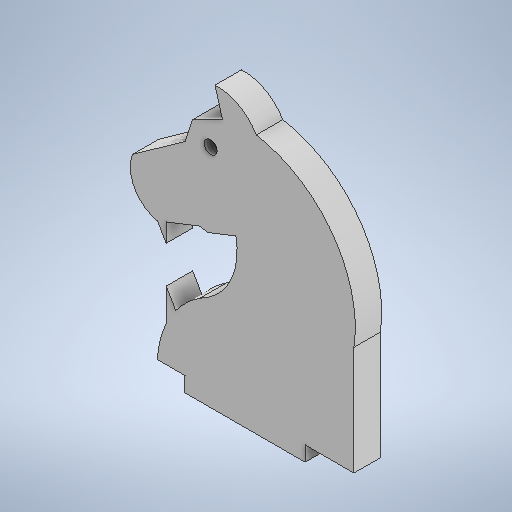
# Autodesk Inventor part: KIGTH TOP ABREBOTELLA 1.2
Saved by Autodesk Inventor 2025.1 (Build 291241000, 241)
## iProperties
Created: 2024-10-24
Part Number: KIGTH TOP ABREBOTELLA 1.2
Material: Genérico
Document SubType Name: Modeling
Designer: Octavio
Density: 1 g/cm^3
Appearance: Valor por defecto
Author: Octavio
Autodesk Inventor part; units mm, degrees
ref_plane "YZ Plane" through (0, 0, 0) normal (1, 0, 0) x (0, 1, 0)
ref_plane "XZ Plane" through (0, 0, 0) normal (0, 1, 0) x (-1, 0, 0)
ref_plane "XY Plane" through (0, 0, 0) normal (0, 0, 1) x (1, 0, 0)
sketch "Boceto1" plane through (0, 0, 0) normal (0, 0, 1) x (1, 0, 0)
  line L0 (-99.9787, 124.5276) -> (102.7005, 124.5276) construction
  line L1 (102.7005, 124.5276) -> (102.7005, -74.7737) construction
  line L2 (102.7005, -74.7737) -> (-99.9787, -74.7737) construction
  line L3 (-99.9787, -74.7737) -> (-99.9787, 124.5276) construction
  line L4 (-22.7001, 0) -> (22.7001, 0)
  line L5 (22.7001, 0) -> (22.7001, 5.675)
  line L6 (22.7001, 5.675) -> (41.1439, 5.675)
  line L7 (41.1439, 5.675) -> (41.1439, 46.8189)
  arc A0 (41.1439, 46.8189) -> (4.2563, 97.8941) centre (-3.4604, 53.4628) ccw
  arc A1 (4.2563, 97.8941) -> (-11.35, 106.4066) centre (-10.6407, 89.1451) ccw
  line L8 (-11.35, 106.4066) -> (-8.5125, 96.4753)
  line L9 (-8.5125, 96.4753) -> (-19.8626, 90.8003)
  line L10 (-19.8626, 90.8003) -> (-22.7001, 82.2878)
  line L11 (-22.7001, 82.2878) -> (-42.5626, 68.1002)
  arc A2 (-42.5626, 68.1002) -> (-33.1043, 51.0752) centre (-30.553, 63.6324) ccw
  line L12 (-33.1043, 51.0752) -> (-17.0251, 57.4095)
  line L13 (-17.0251, 57.4095) -> (-14.1875, 56.7502)
  line L14 (-14.1875, 56.7502) -> (-3.4604, 60.9761)
  arc A3 (-17.0251, 33.8343) -> (-13.8253, 35.6951) centre (-27.9119, 56.2357) ccw
  arc A4 (-17.0251, 33.8343) -> (-22.7001, 29.2293) centre (2.4367, 4.0511) ccw
  line L15 (-33.1043, 5.675) -> (-22.7001, 5.675)
  line L16 (-22.7001, 5.675) -> (-22.7001, 0)
  arc A5 (-22.7001, 29.2293) -> (-30.541, 17.4029) centre (2.4367, 4.0511) ccw
  arc A6 (-30.541, 17.4029) -> (-33.1043, 5.675) centre (2.4367, 4.0511) ccw
  arc A7 (-13.8253, 35.6951) -> (-3.0908, 54.1719) centre (-27.9119, 56.2357) ccw
  arc A8 (-3.0908, 54.1719) -> (-3.4604, 60.9761) centre (-27.9119, 56.2357) ccw
  line L17 (-33.1043, 51.0752) -> (-29.7938, 45.4001)
  line L18 (-29.7938, 45.4001) -> (-29.7938, 52.3793)
  line L19 (-29.7938, 23.7109) -> (-29.7938, 31.4001)
  line L20 (-29.7938, 31.4001) -> (-26.1753, 25.197)
  line L21 (-29.7938, 23.7109) -> (-29.7938, 19.1173)
  point P0 (0, 0)
  dimension "d9" = 14
  constraints: 36 end point, 22 point on circle, 9 centre point, 6 point on line, 4 perpendicular, 2 horizontal, 2 parallel, 1 vertical, 2 other
  measures "d9" distance of L19.end L17.end
extrude "Extrusión1" add sketch "Boceto1" along normal mid plane 10
sketch "Boceto3" plane through (0, 0, 5) normal (0, 0, 1) x (1, 0, 0)
  point P0 (0, 0)
  point P1 (-13.0086, 85.2614)
hole "Agujero2" at (-13.0086, 85.2614, 5) direction (0, 0, -1) diameter 4.917 end through all thread size "M6x1" class "6H" standard "ISO Metric profile"
